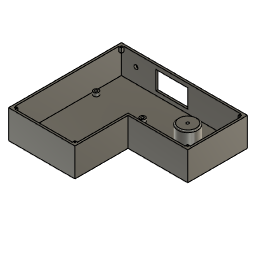
soldeerstation v5 (Autodesk Fusion 360 design; units mm, degrees)
Autodesk Fusion 360 part; units mm, degrees
note: some values were not read from the file. Set by a fixed rule: which sketch regions a step uses.
sketch "Sketch1" plane through (0, 0, 0) normal (0, 0, 1) x (1, 0, 0)
  line L0 (-100, 90) -> (0, 90)
  line L1 (0, 90) -> (0, -80)
  line L2 (0, -80) -> (-100, -80)
  line L3 (-100, -80) -> (-100, 90)
  line L4 (0, 90) -> (90, 90)
  line L5 (90, 90) -> (90, 0)
  line L6 (90, 0) -> (0, 0)
  line L7 (0, 0) -> (0, 90)
  dimension "d1" = 100
  dimension "d2" = 170
  dimension "d3" = 90
  dimension "d4" = 90
  constraint horizontal L0
  constraint vertical L1
  constraint horizontal L2
  constraint vertical L3
  constraint horizontal L4
  constraint vertical L5
  constraint horizontal L6
  constraint vertical L7
  constraint coincident L6.end L7.start
  measures "d1" distance of L0.start L0.end
  measures "d2" distance of L0.start L2.end
  measures "d3" distance of L0.end L4.end
  measures "d4" distance of L4.end L5.end
extrude "Extrude1" add sketch "Sketch1" along normal blind 3
sketch "Sketch2" plane through (0, 0, 3) normal (0, 0, 1) x (-1, 0, 0)
  line L0 (-90, 0) -> (-90, -90)
  line L1 (-90, -90) -> (100, -90)
  line L2 (100, -90) -> (100, 80)
  line L3 (100, 80) -> (0, 80)
  line L4 (0, 80) -> (0, 0)
  line L5 (0, 0) -> (-90, 0)
  line L6 (97, -87) -> (3, -87)
  line L7 (3, -87) -> (3, 77)
  line L8 (3, 77) -> (97, 77)
  line L9 (97, 77) -> (97, -87)
  line L10 (3, -87) -> (-87, -87)
  line L11 (-87, -87) -> (-87, -3)
  line L12 (-87, -3) -> (3, -3)
  line L13 (3, -3) -> (3, -87)
  dimension "d7" = 3
  dimension "d8" = 3
  dimension "d9" = 3
  dimension "d10" = 3
  dimension "d12" = 97
  dimension "d13" = 3
  constraint horizontal L6
  constraint vertical L7
  constraint horizontal L8
  constraint vertical L9
  constraint horizontal L10
  constraint vertical L11
  constraint horizontal L12
  constraint vertical L13
  measures "d7" distance of L5 L12
  measures "d8" distance of L0 L11
  measures "d9" distance of L1 L10
  measures "d10" distance of L2 L9
  measures "d12" distance of L2 L7
  measures "d13" distance of L3 L8
extrude "Extrude2" add sketch "Sketch2" along normal blind 40
sketch "Sketch3" plane through (0, 0, 3) normal (0, 0, 1) x (-1, 0, 0)
  line L0 (-87, -87) -> (97, -87)
  line L1 (97, -87) -> (97, 77)
  line L2 (97, 77) -> (3, 77)
  line L3 (3, 77) -> (3, -3)
  line L4 (3, -3) -> (-87, -3)
  line L5 (-87, -3) -> (-87, -87)
  circle A0 centre (-45, -45) radius 15
  line L6 (-90, -90) -> (100, -90)
  line L7 (-90, 0) -> (-90, -90)
  dimension "d16" = 30
  dimension "d17" = 45
  dimension "d18" = 45
  measures "d16" diameter of A0
  measures "d17" distance of A0.centre L6
  measures "d18" distance of A0.centre L7
extrude "Extrude3" add sketch "Sketch3" along normal blind 30 contours A0
sketch "Sketch4" plane through (0, 0, 33) normal (0, 0, 1) x (-1, 0, 0)
  circle A0 centre (-45, -45) radius 15
  circle A1 centre (-45, -45) radius 2
  dimension "d21" = 4
  constraint concentric A0 A1
  measures "d21" diameter of A1
extrude "Extrude4" cut sketch "Sketch4" against normal blind 30 contours A1
fillet "Fillet1" radius 2 1 edges at (58.9849, 50.4242, 33)
sketch "Sketch5" plane through (-97, 0, 0) normal (1, 0, 0) x (0, 1, 0)
  line L0 (-77, 3) -> (87, 3)
  line L1 (87, 3) -> (87, 43)
  line L2 (87, 43) -> (-77, 43)
  line L3 (-77, 43) -> (-77, 3)
  line L4 (87, 43) -> (83, 43)
  line L5 (83, 43) -> (83, 36)
  line L6 (83, 36) -> (87, 36)
  line L7 (87, 36) -> (87, 43)
  dimension "d26" = 4
  dimension "d27" = 7
  constraint horizontal L4
  constraint vertical L5
  constraint horizontal L6
  constraint vertical L7
  constraint coincident L1.end L2.start
  measures "d26" distance of L5 L7
  measures "d27" distance of L4 L6
extrude "Extrude5" add sketch "Sketch5" along normal blind 4 contours L1 L2 L4 L5 L6 L7
sketch "Sketch6" plane through (0, 0, 43) normal (0, 0, 1) x (-1, 0, 0)
  line L0 (-87, -87) -> (-87, -3)
  line L1 (-87, -3) -> (3, -3)
  line L2 (3, -3) -> (3, 77)
  line L3 (3, 77) -> (97, 77)
  line L4 (97, 77) -> (97, -83)
  line L5 (97, -83) -> (93, -83)
  line L6 (93, -83) -> (93, -87)
  line L7 (93, -87) -> (-87, -87)
  line L8 (0, 0) -> (-90, 0)
  line L9 (-90, 0) -> (-90, -90)
  line L10 (-90, -90) -> (100, -90)
  line L11 (100, -90) -> (100, 80)
  line L12 (100, 80) -> (0, 80)
  line L13 (0, 80) -> (0, 0)
  line L14 (3, 77) -> (7, 77)
  line L15 (7, 77) -> (7, 73)
  line L16 (7, 73) -> (3, 73)
  line L17 (3, 73) -> (3, 77)
  line L18 (97, 77) -> (93, 77)
  line L19 (93, 77) -> (93, 73)
  line L20 (93, 73) -> (97, 73)
  line L21 (97, 73) -> (97, 77)
  line L22 (-87, -87) -> (-83, -87)
  line L23 (-83, -87) -> (-83, -83)
  line L24 (-83, -83) -> (-87, -83)
  line L25 (-87, -83) -> (-87, -87)
  line L26 (-87, -3) -> (-83, -3)
  line L27 (-83, -3) -> (-83, -7)
  line L28 (-83, -7) -> (-87, -7)
  line L29 (-87, -7) -> (-87, -3)
  circle A0 centre (-85, -5) radius 1.1
  circle A1 centre (-85, -85) radius 1.1
  circle A2 centre (5, 75) radius 1.1
  circle A3 centre (95, 75) radius 1.1
  dimension "d30" = 4
  dimension "d31" = 4
  dimension "d32" = 4
  dimension "d33" = 4
  dimension "d34" = 4
  dimension "d35" = 4
  dimension "d36" = 4
  dimension "d37" = 4
  dimension "d38" = 2.2
  dimension "d39" = 2
  dimension "d40" = 2
  dimension "d41" = 2.2
  dimension "d42" = 2
  dimension "d43" = 2
  dimension "d44" = 2.2
  dimension "d45" = 2
  dimension "d46" = 2
  dimension "d47" = 2.2
  dimension "d48" = 2
  dimension "d49" = 2
  constraint horizontal L14
  constraint vertical L15
  constraint horizontal L16
  constraint vertical L17
  constraint coincident L2.end L3.start
  constraint horizontal L18
  constraint vertical L19
  constraint horizontal L20
  constraint vertical L21
  constraint coincident L3.end L4.start
  constraint horizontal L22
  constraint vertical L23
  constraint horizontal L24
  constraint vertical L25
  constraint coincident L0.start L7.end
  constraint horizontal L26
  constraint vertical L27
  constraint horizontal L28
  constraint vertical L29
  constraint coincident L0.end L1.start
  measures "d30" distance of L27 L29
  measures "d31" distance of L26 L28
  measures "d32" distance of L14 L16
  measures "d33" distance of L15.end L16.end
  measures "d34" distance of L19.end L20.end
  measures "d35" distance of L18.end L19.end
  measures "d36" distance of L23.end L24.end
  measures "d37" distance of L22.end L23.end
  measures "d38" diameter of A0
  measures "d39" distance of L27 A0.centre
  measures "d40" distance of L28 A0.centre
  measures "d41" diameter of A1
  measures "d42" distance of L23 A1.centre
  measures "d43" distance of L24 A1.centre
  measures "d44" diameter of A2
  measures "d45" distance of L15 A2.centre
  measures "d46" distance of L16 A2.centre
  measures "d47" diameter of A3
  measures "d48" distance of L19 A3.centre
  measures "d49" distance of L20 A3.centre
extrude "Extrude6" add sketch "Sketch6" against normal blind 7 contours L0 L7 L22 L23 L24 L25 | L0 L1 L26 L27 L28 L29 | L3 L4 L18 L19 L20 L21 | L2 L3 L14 L15 L16 L17
sketch "Sketch7" plane through (0, 0, 43) normal (0, 0, 1) x (-1, 0, 0)
  circle A0 centre (-85, -85) radius 1.1
  circle A1 centre (5, 75) radius 1.1
  circle A2 centre (-85, -5) radius 1.1
  circle A3 centre (95, 75) radius 1.1
  line L0 (-87, -83) -> (-87, -7)
  line L1 (-87, -7) -> (-83, -7)
  line L2 (-83, -7) -> (-83, -3)
  line L3 (-83, -3) -> (3, -3)
  line L4 (3, -3) -> (3, 73)
  line L5 (3, 73) -> (7, 73)
  line L6 (7, 73) -> (7, 77)
  line L7 (7, 77) -> (93, 77)
  line L8 (93, 77) -> (93, 73)
  line L9 (93, 73) -> (97, 73)
  line L10 (97, 73) -> (97, -83)
  line L11 (97, -83) -> (93, -83)
  line L12 (93, -83) -> (93, -87)
  line L13 (93, -87) -> (-83, -87)
  line L14 (-83, -87) -> (-83, -83)
  line L15 (-83, -83) -> (-87, -83)
  line L16 (0, 0) -> (-90, 0)
  line L17 (-90, 0) -> (-90, -90)
  line L18 (-90, -90) -> (100, -90)
  line L19 (100, -90) -> (100, 80)
  line L20 (100, 80) -> (0, 80)
  line L21 (0, 80) -> (0, 0)
  circle A4 centre (95, -85) radius 1.1
  dimension "d52" = 2.2
  dimension "d53" = 2
  dimension "d54" = 2
  measures "d52" diameter of A4
  measures "d53" distance of L12 A4.centre
  measures "d54" distance of L11 A4.centre
extrude "Extrude7" cut sketch "Sketch7" against normal blind 7 contours A4
sketch "Sketch8" plane through (0, 90, 0) normal (0, 1, 0) x (-1, 0, 0)
  line L0 (-90, 0) -> (100, 0)
  line L1 (100, 0) -> (100, 43)
  line L2 (100, 43) -> (-90, 43)
  line L3 (-90, 43) -> (-90, 0)
  line L4 (-3, 37) -> (45, 37)
  line L5 (45, 37) -> (45, 9)
  line L6 (45, 9) -> (-3, 9)
  line L7 (-3, 9) -> (-3, 37)
  dimension "d57" = 48
  dimension "d58" = 28
  dimension "d59" = 55
  dimension "d60" = 6
  constraint horizontal L4
  constraint vertical L5
  constraint horizontal L6
  constraint vertical L7
  measures "d57" distance of L5 L7
  measures "d58" distance of L4 L6
  measures "d59" distance of L1 L5
  measures "d60" distance of L2 L4
extrude "Extrude8" cut sketch "Sketch8" against normal blind 3 contours L4 L5 L6 L7
sketch "Sketch9" plane through (0, 0, 3) normal (0, 0, 1) x (-1, 0, 0)
  circle A0 centre (-45, -45) radius 15
  line L0 (-87, -87) -> (97, -87)
  line L1 (97, -87) -> (97, 77)
  line L2 (97, 77) -> (3, 77)
  line L3 (3, 77) -> (3, -3)
  line L4 (3, -3) -> (-87, -3)
  line L5 (-87, -3) -> (-87, -87)
  line L6 (21, 71) -> (91, 71)
  line L7 (91, 71) -> (91, -43)
  line L8 (91, -43) -> (21, -43)
  line L9 (21, -43) -> (21, 71)
  circle A1 centre (21, 71) radius 4
  circle A2 centre (91, 71) radius 4
  circle A3 centre (21, -43) radius 4
  circle A4 centre (91, -43) radius 4
  circle A5 centre (91, -43) radius 1.9
  circle A6 centre (21, -43) radius 1.9
  circle A7 centre (91, 71) radius 1.9
  circle A8 centre (21, 71) radius 1.9
  dimension "d63" = 70
  dimension "d64" = 114
  dimension "d65" = 6
  dimension "d66" = 6
  dimension "d67" = 8
  dimension "d68" = 8
  dimension "d69" = 8
  dimension "d70" = 8
  dimension "d79" = 3.8
  dimension "d80" = 3.8
  dimension "d81" = 3.8
  dimension "d82" = 3.8
  constraint horizontal L6
  constraint vertical L7
  constraint horizontal L8
  constraint vertical L9
  constraint coincident L6.start L9.end
  constraint coincident L6.end L7.start
  constraint coincident L8.end L9.start
  constraint coincident L7.end L8.start
  constraint concentric A4 A5
  constraint concentric A3 A6
  constraint concentric A2 A7
  constraint concentric A1 A8
  measures "d63" distance of L7 L9
  measures "d64" distance of L6.start L8.end
  measures "d65" distance of L1 L7
  measures "d66" distance of L2 L6
  measures "d67" diameter of A1
  measures "d68" diameter of A2
  measures "d69" diameter of A3
  measures "d70" diameter of A4
  measures "d79" diameter of A5
  measures "d80" diameter of A6
  measures "d81" diameter of A7
  measures "d82" diameter of A8
extrude "Extrude9" add sketch "Sketch9" along normal blind 5 contours L6 L9 A8 | L6 L9 A8 | L6 L9 A1 A8 | L6 L9 A1 A8 | L6 L7 A2 A7 | L6 L7 A2 A7 | L8 L9 A3 A6 | L8 L9 A3 A6 | L6 L7 A7 | L6 L7 A7 | L8 L9 A6 | L8 L9 A6 | L7 L8 A4 A5 | L7 L8 A4 A5 | L7 L8 A5 | L7 L8 A5
sketch "Sketch10" plane through (0, 0, 8) normal (0, 0, 1) x (-1, 0, 0)
  circle A0 centre (21, 71) radius 4
  circle A1 centre (21, 71) radius 1.8
  circle A2 centre (91, 51) radius 1.8
  circle A3 centre (91, -63) radius 1.8
  circle A4 centre (27, -63) radius 1.8
  dimension "d73" = 3.6
  dimension "d74" = 3.6
  dimension "d75" = 3.6
  dimension "d76" = 3.6
  constraint concentric A0 A1
  measures "d73" diameter of A1
  measures "d74" diameter of A2
  measures "d75" diameter of A3
  measures "d76" diameter of A4
extrude "Extrude10" cut sketch "Sketch10" against normal blind 5 contours A1 | A2 | A3 | A4
sketch "Sketch11" plane through (0, 0, 8) normal (0, 0, 1) x (-1, 0, 0)
  circle A0 centre (21, -43) radius 4
  circle A1 centre (21, -43) radius 1.9
  circle A2 centre (91, -43) radius 1.9
  circle A3 centre (91, -43) radius 4
  circle A4 centre (91, 71) radius 1.9
  circle A5 centre (91, 71) radius 4
  dimension "d83" = 3.8
  dimension "d84" = 3.8
  dimension "d85" = 3.8
  constraint concentric A0 A1
  constraint concentric A2 A3
  constraint concentric A4 A5
  measures "d83" diameter of A1
  measures "d84" diameter of A2
  measures "d85" diameter of A4
extrude "Extrude11" cut sketch "Sketch11" against normal blind 5 contours A1 | A2 | A4
sketch "Sketch12" plane through (0, 90, 0) normal (0, 1, 0) x (-1, 0, 0)
  line L0 (45, 37) -> (45, 9)
  line L1 (45, 9) -> (-3, 9)
  line L2 (-3, 9) -> (-3, 37)
  line L3 (-3, 37) -> (45, 37)
  line L4 (-90, 0) -> (100, 0)
  line L5 (100, 0) -> (100, 43)
  line L6 (100, 43) -> (-90, 43)
  line L7 (-90, 43) -> (-90, 0)
  circle A0 centre (75, 25) radius 3
  dimension "d88" = 6
  measures "d88" diameter of A0
extrude "Extrude12" cut sketch "Sketch12" against normal blind 3 contours A0
